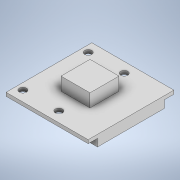
# Autodesk Inventor part: Camera
Saved by Autodesk Inventor 2020 (Build 240168000, 168)
## iProperties
Created: 2019-09-04
Part Number: Camera
Material: Generic
Document SubType Name: Modeling
Designer: User
Density: 1 g/cm^3
Appearance: Default
Author: User
Autodesk Inventor part; units mm, degrees
ref_plane "YZ Plane" through (0, 0, 0) normal (1, 0, 0) x (0, 1, 0)
ref_plane "XZ Plane" through (0, 0, 0) normal (0, 1, 0) x (-1, 0, 0)
ref_plane "XY Plane" through (0, 0, 0) normal (0, 0, 1) x (1, 0, 0)
sketch "Sketch1" plane through (0, 0, 0) normal (0, 1, 0) x (-1, 0, 0)
  line L0 (-11.9316, 12.465) -> (11.9317, 12.465)
  line L1 (11.9317, 12.465) -> (11.9316, -12.465)
  line L2 (11.9316, -12.465) -> (-11.9317, -12.465)
  line L3 (-11.9317, -12.465) -> (-11.9316, 12.465)
  line L4 (-11.9316, 12.465) -> (11.9316, -12.465) construction
  line L5 (11.9317, 12.465) -> (-11.9317, -12.465) construction
  circle A0 centre (10.0076, 9.4933) radius 1.0351
  line L6 (0, 0) -> (10.0076, 0) construction
  line L7 (10.0076, 0) -> (10.0076, 9.4933) construction
  line L8 (4.7752, 0) -> (4.7752, 3.1605) construction
  circle A1 centre (10.0076, -9.4933) radius 1.0351
  circle A2 centre (-0.4572, 9.4933) radius 1.0351
  circle A3 centre (-0.4572, -9.4933) radius 1.0351
  dimension "d0" = 24.9301
  dimension "d1" = 23.8633
  dimension "d2" = 2.0701
  dimension "d3" = 1.9241
  dimension "d5" = 5.2324
  dimension "d16" = 18.9865
  constraints: 18 end point, 4 centre point, 3 symmetric about line, 2 horizontal, 2 midpoint, 2 parallel, 2 perpendicular, 1 point on line, 1 vertical, 3 other
  measures "d0" distance of L2.end L0.start
  measures "d1" distance of L0.start L0.end
  measures "d2" diameter of A0
  measures "d3" distance between parallel lines of L1 L7
  measures "d5" distance between parallel lines of L8 L7
  measures "d16" distance of L7.end A1.centre
extrude "Extrusion1" add sketch "Sketch1" along normal blind 1.016
sketch "Sketch2" plane through (0, 1.016, 0) normal (0, 1, 0) x (1, 0, 0)
  line L0 (4.2101, -4.21) -> (-4.21, -4.21)
  line L1 (-4.21, -4.21) -> (-4.21, 4.21)
  line L2 (-4.21, 4.21) -> (4.2101, 4.2101)
  line L3 (4.2101, 4.2101) -> (4.2101, -4.21)
  line L4 (4.2101, -4.21) -> (-4.21, 4.21) construction
  line L5 (-4.21, -4.21) -> (4.2101, 4.2101) construction
  point P0 (0, 0)
  dimension "d8" = 8.4201
  dimension "d9" = 8.4201
  constraints: 12 end point, 2 midpoint, 2 parallel, 1 horizontal, 1 perpendicular
  measures "d8" distance of L0.end L1.end
  measures "d9" distance of L1.end L2.end
extrude "Extrusion2" add sketch "Sketch2" along normal blind 3.81
sketch "Sketch3" plane through (0, 0, 0) normal (0, -1, 0) x (1, 0, 0)
  line L0 (11.9316, 12.465) -> (11.9317, -12.465) projected
  line L1 (6.5977, 9.7536) -> (11.9317, 9.7536)
  line L2 (11.9317, 9.7536) -> (11.9317, -9.7536)
  line L3 (11.9317, -9.7536) -> (6.5977, -9.7536)
  line L4 (6.5977, -9.7536) -> (6.5977, 9.7536)
  line L5 (6.5977, 9.7536) -> (11.9317, -9.7536) construction
  line L6 (11.9317, 9.7536) -> (6.5977, -9.7536) construction
  line L7 (0, 0) -> (9.2647, 0) construction
  dimension "d12" = 5.334
  dimension "d13" = 19.5072
  constraints: 14 end point, 2 midpoint, 2 parallel, 2 perpendicular, 1 horizontal, 1 point on line
  measures "d12" distance between parallel lines of L0 L4
  measures "d13" distance between parallel lines of L1 L3
extrude "Extrusion3" add sketch "Sketch3" along normal blind 2.1844
body "Solid1"
